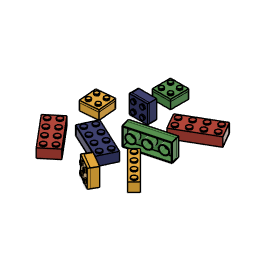
Lego v7 (Autodesk Fusion 360 design; units mm, degrees)
Autodesk Fusion 360 part; units mm, degrees
note: some values were not read from the file. Set by a fixed rule: which face or edge a step refers to.
sketch "Sketch1" plane through (0, 0, 0) normal (0, 1, 0) x (1, 0, 0)
  line L0 (-45, 20) -> (45, 20)
  line L1 (45, 20) -> (45, -20)
  line L2 (45, -20) -> (-45, -20)
  line L3 (-45, -20) -> (-45, 20)
  dimension "d12" = 20
  dimension "d13" = 20
  dimension "d32" = 45
  dimension "d33" = 45
  constraint horizontal L0
  constraint perpendicular L0 L1
  constraint parallel L0 L2
  constraint parallel L1 L3
  measures "d12" distance of L0 origin
  measures "d13" distance of origin L2
  measures "d32" distance of origin L3
  measures "d33" distance of origin L1
extrude "Extrude1" add sketch "Sketch1" along normal blind 20 makes body 1
sketch "Sketch2" plane through (0, 20, 0) normal (0, 1, 0) x (-1, 0, 0)
  line L0 (45, 20) -> (-45, 20)
  line L1 (-45, 20) -> (-45, -20)
  line L2 (-45, -20) -> (45, -20)
  line L3 (45, -20) -> (45, 20)
  circle A0 centre (35, -10) radius 6
  circle A1 centre (11.6667, -10) radius 6
  circle A2 centre (-11.6667, -10) radius 6
  circle A3 centre (-35, -10) radius 6
  line L4 (0, 0) -> (-59, 0) construction
  line L5 (0, 0) -> (56, 0) construction
  circle A4 centre (-35, 10) radius 6
  circle A5 centre (-11.6667, 10) radius 6
  circle A6 centre (35, 10) radius 6
  circle A7 centre (11.6667, 10) radius 6
  dimension "d5" = -70
  dimension "d6" = 28
  dimension "d15" = 10
  dimension "d16" = 12
  constraint coincident L4.start L5.start
  constraint perpendicular L1 L4
  constraint perpendicular L3 L5
  constraint symmetric A0 L4 A6
  constraint symmetric A1 L4 A7
  constraint symmetric A2 L4 A5
  constraint symmetric A3 L4 A4
  measures "d15" vertical distance of L4.start A0.centre
  measures "d16" diameter of A0
extrude "Extrude2" add sketch "Sketch2" along normal blind 2 contours A0 | A1 | A2 | A3 | A4 | A5 | A6 | A7 bodies 1
fillet "Fillet1" radius 0.4 8 faces at (10.2006, 22, -8.0435) (-13.8354, 22, -11.4247) (-34.8505, 22, -8.0947) (38.439, 22, -9.7019) (-36.8505, 22, 8.0056) (-10.6667, 22, 11.7321) (12.4909, 22, 7.1021) (36.0263, 22, 11.9063) on bodies 1
sketch "Sketch3" plane through (0, 0, 0) normal (0, -1, 0) x (1, 0, 0)
  line L0 (45, 20) -> (-45, 20)
  line L1 (-45, 20) -> (-45, -20)
  line L2 (-45, -20) -> (45, -20)
  line L3 (45, -20) -> (45, 20)
  line L4 (-43.3751, 18.3751) -> (-43.3751, -18.3751)
  line L5 (-43.3751, -18.3751) -> (43.3751, -18.3751)
  line L6 (43.3751, -18.3751) -> (43.3751, 18.3751)
  line L7 (43.3751, 18.3751) -> (-43.3751, 18.3751)
  dimension "d17" = -1.6249
extrude "Extrude3" cut sketch "Sketch3" against normal blind 15 contours L4 L5 L6 L7 bodies 1
sketch "Sketch4" plane through (0, 15, 0) normal (0, -1, 0) x (1, 0, 0)
  line L0 (43.3751, 18.3751) -> (-43.3751, 18.3751)
  line L1 (-43.3751, 18.3751) -> (-43.3751, -18.3751)
  line L2 (-43.3751, -18.3751) -> (43.3751, -18.3751)
  line L3 (43.3751, -18.3751) -> (43.3751, 18.3751)
  line L4 (0, 30) -> (0, -35) construction
  circle A0 centre (0, 0) radius 10
  circle A1 centre (-30, 0) radius 10
  circle A2 centre (30, 0) radius 10
  circle A3 centre (0, 0) radius 8.8122
  circle A4 centre (-30, 0) radius 8.8122
  circle A5 centre (30, 0) radius 8.8122
  dimension "d20" = 20
  dimension "d23" = 30
  dimension "d24" = 0
  dimension "d25" = -1.1878
  dimension "d28" = 30
  dimension "d29" = 0
  constraint perpendicular L2 L4
  constraint coincident A0.centre A3.centre
  measures "d20" diameter of A0
extrude "Extrude4" add sketch "Sketch4" along normal up to surface (15 mm away) contours A0 | A1 | A2 bodies 1
copy_body "CopyPasteBodies1" bodies 1 makes body 2
copy_body "CopyPasteBodies2" bodies 2 makes body 3
copy_body "CopyPasteBodies3" bodies 3 makes body 4
copy_body "CopyPasteBodies4" bodies 4 makes body 5
move_body "Move1" bodies 1 to x (0.906308, 0, 0.422618) y (0, 1, 0) z (-0.422618, 0, 0.906308) at (0, 0, 80)
move_body "Move2" bodies 3 to x (0.642788, 0, 0.766044) y (0, 1, 0) z (-0.766044, 0, 0.642788) at (-62.4663, 0, 118.5883)
move_body "Move3" bodies 4 to x (0.866025, 0, -0.5) y (0, 1, 0) z (0.5, 0, 0.866025) at (0, 0, -70)
move_body "Move4" bodies 5 to x (0.965926, 0, -0.258819) y (-0.258819, 0, -0.965926) z (0, 1, 0) at (125.1764, 20, 19.3185)
move_body "Move5" bodies 2 to x (0.707107, 0, 0.707107) y (0, 1, 0) z (-0.707107, 0, 0.707107) at (142.988, 0, 80.1646)
sketch "Sketch5" plane through (0, 20, 0) normal (0, 1, 0) x (-1, 0, 0)
  circle A0 centre (-160.6657, 111.9844) radius 6
  circle A1 centre (-125.3104, 48.3448) radius 6
  circle A2 centre (-174.8078, 97.8423) radius 6
  circle A3 centre (-111.1682, 62.4869) radius 6
  circle A4 centre (-144.1665, 95.4852) radius 6
  circle A5 centre (-141.8095, 64.8439) radius 6
  circle A6 centre (-158.3087, 81.3431) radius 6
  circle A7 centre (-127.6674, 78.9861) radius 6
  line L0 (-97.0261, 62.4869) -> (-160.6657, 126.1265)
  line L1 (-160.6657, 126.1265) -> (-188.95, 97.8423)
  line L2 (-188.95, 97.8423) -> (-125.3104, 34.2027)
  line L3 (-125.3104, 34.2027) -> (-97.0261, 62.4869)
  line L4 (-174.8078, 111.9844) -> (-111.1682, 48.3448)
  constraint midpoint L1 L4.start
  constraint midpoint L3 L4.end
split "Split1" by curves path "Sketch5" along L4 bodies 2 makes body 6 at (146.5236, 6.6667, 55.4159)
delete_body "RemoveBody1" bodies 2
sketch "Sketch6" plane through (0, 0, 0) normal (0, 1, 0) x (1, 0, 0)
  line L0 (-20, 20) -> (20, 20)
  line L1 (20, 20) -> (20, -20)
  line L2 (20, -20) -> (-20, -20)
  line L3 (-20, -20) -> (-20, 20)
  line L4 (-19, -19) -> (-19, 19)
  line L5 (-19, 19) -> (19, 19)
  line L6 (19, 19) -> (19, -19)
  line L7 (19, -19) -> (-19, -19)
  line L8 (0, 14) -> (0, 0) construction
  line L9 (0, 0) -> (-15, 0) construction
  circle A0 centre (-10, 10) radius 5
  circle A1 centre (10, 10) radius 5
  circle A2 centre (-10, -10) radius 5
  circle A3 centre (10, -10) radius 5
  circle A4 centre (0, 0) radius 5
  circle A5 centre (0, 0) radius 4.3804
  dimension "d46" = 1
  dimension "d47" = 10
  dimension "d48" = 10
  dimension "d49" = -0.6196
  constraint horizontal L0
  constraint perpendicular L0 L1
  constraint parallel L0 L2
  constraint parallel L1 L3
  constraint coincident L8.end L9.start
  constraint vertical L8
  constraint perpendicular L8 L9
  constraint symmetric L8 A0 A1
  constraint symmetric L9 A0 A2
  constraint symmetric L9 A1 A3
  measures "d47" diameter of A0
  measures "d48" diameter of A4
extrude "Extrude5" add sketch "Sketch6" along normal blind 20 separate body contours L0 L1 L2 L3 makes body 7
extrude "Extrude6" add sketch "Sketch6" against normal blind 5 from surface at 20 contours L4 L5 L6 L7 | A0 | A1 | A2 | A3 | A4 | A5 bodies 7
extrude "Extrude7" add sketch "Sketch6" along normal blind 3 from surface at 20 contours A0 | A1 | A2 | A3 bodies 7
extrude "Extrude8" add sketch "Sketch6" along normal up to surface (15 mm away) contours A4 bodies 7
copy_body "CutPasteBodies1" bodies 1 6 5 4 3 removing the originals makes body 8 makes body 9 makes body 10 makes body 11 makes body 12 in component "rectangle"
fillet "Fillet2" radius 0.5 4 edges at (-14.6616, 23, 11.8081) (-14.6616, 23, -8.1919) (5.3384, 23, -8.1919) (5.3384, 23, 11.8081) on bodies 7
copy_body "CopyPasteBodies5" bodies 7 makes body 13
copy_body "CopyPasteBodies6" bodies 13 7 makes body 14 makes body 15
move_body "Move1'" bodies 11 to x (1, 0, 0) y (0, 1, 0) z (0, 0, 1) at (86.4357, 0, 15.0708) in component "rectangle"
move_body "Move6" bodies 7 to x (1, 0, 0) y (0, 1, 0) z (0, 0, 1) at (-13.7411, 0, -64.2727)
move_body "Move7" bodies 14 to x (0.996195, 0, -0.087156) y (0, 1, 0) z (0.087156, 0, 0.996195) at (-73.8146, 0, 6.3096)
move_body "Move8" bodies 15 to x (1, 0, 0) y (0, 1, 0) z (0, 0, 1) at (56.5145, 0, 145.9312)
move_body "Move2'" bodies 9 10 to x (1, 0, 0) y (0, 1, 0) z (0, 0, 1) at (-58.0628, 0, 18.5801) in component "rectangle"
move_body "Move9" bodies 15 to x (0.866025, 0, 0.5) y (-0.5, 0, 0.866025) z (0, -1, 0) at (10.0715, 165.9312, 113.3438)
move_body "Move10" bodies 13 to x (1, 0, 0) y (0, 0, 1) z (0, -1, 0) at (-10, 20, -40)
move_body "Move11" bodies 7 to x (1, 0, 0) y (0, 1, 0) z (0, 0, 1) at (0, 0, -30)
component "rectangle" placed x (1, 0, 0) y (0, 1, 0) z (0, 0, 1) at (0, 0, 0)
